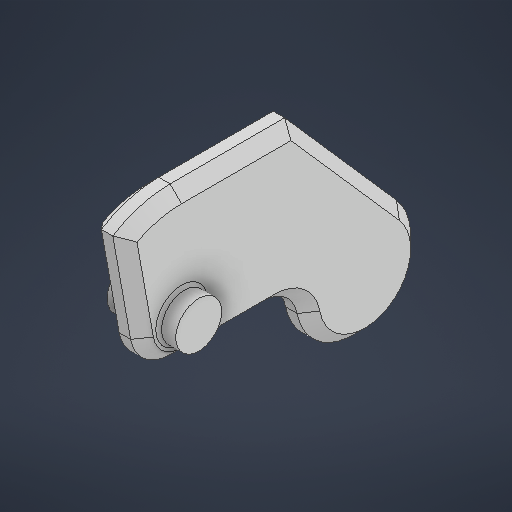
# Autodesk Inventor part: TrainPullert
Saved by Autodesk Inventor 2026.3 (Build 303398000, 398)
## iProperties
Created: 2026-05-02
Part Number: TrainPullert
Material: Generic
Document SubType Name: Modeling
Designer: frede
Density: 1 g/cm^3
Appearance: Default
Author: frede
Autodesk Inventor part; units mm, degrees
ref_plane "YZ Plane" through (0, 0, 0) normal (1, 0, 0) x (0, 1, 0)
ref_plane "XZ Plane" through (0, 0, 0) normal (0, 1, 0) x (-1, 0, 0)
ref_plane "XY Plane" through (0, 0, 0) normal (0, 0, 1) x (1, 0, 0)
sketch "Sketch1" plane through (0, 0, 0) normal (1, 0, 0) x (0, 1, 0)
  arc A0 (9.4, 0) -> (7.9599, 5) centre (0, 0) ccw
  circle A1 centre (0, 0) radius 3.5
  line L0 (-0.6243, 3.4439) -> (7.9599, 5)
  line L1 (-3.5, 0) -> (-3.5, -8.9713)
  line L2 (9.4, 0) -> (9.4, -10)
  line L3 (-3.5, -8.9713) -> (-4.2585, -11.0553)
  line L4 (-3.5, -8.9713) -> (26.5, -8.9713) construction
  line L5 (-1.6991, -19.7555) -> (9.4, -10)
  arc A2 (-4.2585, -11.0553) -> (-1.6991, -19.7555) centre (-5, -16) ccw
  dimension "d0" = 18.8
  dimension "d2" = 7
  dimension "d4" = 5
  dimension "d5" = 10
  dimension "d7" = 110
  dimension "d26" = 10
  dimension "d27" = 5
  dimension "d28" = 16
  constraints: 12 end point, 6 point on circle, 4 tangent, 3 centre point, 2 coincident, 2 vertical, 1 horizontal
  measures "d0" diameter of A0
  measures "d2" diameter of A1
  measures "d4" vertical distance of point (0, 0) L0.end
  measures "d5" distance of L2.start L2.end
  measures "d7" angle of L3 L4
  measures "d26" diameter of A2
  measures "d27" horizontal distance of point (0, 0) A2.centre
  measures "d28" vertical distance of A2.centre point (0, 0)
extrude "Extrusion1" add sketch "Sketch1" along normal blind 3
sketch "Sketch2" plane through (3, 0, 0) normal (1, 0, 0) x (0, 0, -1)
  circle A0 centre (0, 0) radius 2
  dimension "d12" = 4
  constraints: 1 centre point, 1 coincident
  measures "d12" diameter of A0
extrude "Extrusion2" add sketch "Sketch2" along normal blind 1.5
sketch "Sketch3" plane through (0, 0, 0) normal (-1, 0, 0) x (0, 0, 1)
  circle A0 centre (0, 0) radius 2
  dimension "d15" = 4
  constraints: 1 centre point, 1 coincident
  measures "d15" diameter of A0
extrude "Extrusion3" add sketch "Sketch3" along normal blind 1.5
fillet "Fillet2" radius 3 2 edges at (1.5, -4.2585, -11.0553) (1.5, -3.5, -8.9713)
fillet "Fillet1" radius 0.25 2 edges at (3, 0, 2) (0, 0, -2)
chamfer "Chamfer2" distance 1 angle 45 16 edges at (0, 9.4, -5) (0, 9.0328, 2.6016) (3, 9.4, -5) (3, 9.0328, 2.6016) (0, 3.6678, 4.2219) (0, -2.6865, 2.2433) (0, -3.5, -4.0709) (0, -4.1883, -10.054) (0, -9.4917, -18.1966) (0, 3.8505, -14.8778) (3, 3.6678, 4.2219) (3, -2.6865, 2.2433) (3, -3.5, -4.0709) (3, -4.1883, -10.054) (3, -9.4917, -18.1966) (3, 3.8505, -14.8778)
body "Solid1"
